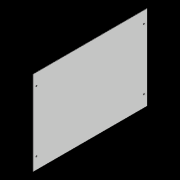
# Autodesk Inventor part: TopV4
Saved by Autodesk Inventor 2022 (Build 260153000, 153)
## iProperties
Created: 2021-10-02
Part Number: TopV4
Material: Generic
Document SubType Name: Modeling
Designer: timmy
Density: 1 g/cm^3
Appearance: Default
Author: timmy
Autodesk Inventor part; units mm, degrees
ref_plane "YZ Plane" through (0, 0, 0) normal (1, 0, 0) x (0, 1, 0)
ref_plane "XZ Plane" through (0, 0, 0) normal (0, 1, 0) x (-1, 0, 0)
ref_plane "XY Plane" through (0, 0, 0) normal (0, 0, 1) x (1, 0, 0)
sketch "Sketch1" plane through (0, 0, 0) normal (1, 0, 0) x (0, 1, 0)
  line L0 (0, 0) -> (383.54, 0)
  line L1 (383.54, 0) -> (383.54, -518.922)
  line L2 (383.54, -518.922) -> (0, -518.922)
  line L3 (0, -518.922) -> (0, 0)
  dimension "d0" = 383.54
  dimension "d1" = 518.922
  constraints: 8 end point, 2 parallel, 1 horizontal, 1 perpendicular
  measures "d0" distance of L1.end L2.end
  measures "d1" distance of L0.end L1.end
extrude "Extrusion1" add sketch "Sketch1" along normal blind 1.5875
sketch "Sketch2" plane through (1.5875, 0, 0) normal (1, 0, 0) x (0, 0, -1)
  line L0 (0, 191.77) -> (105.6706, 191.77)
  line L1 (0, 0) -> (518.922, 0) projected
  line L2 (259.461, 0) -> (259.461, 125.3156)
  line L3 (259.461, 383.54) -> (259.461, 258.2244)
  circle A0 centre (14.986, 53.4416) radius 3.175
  line L4 (518.922, 191.77) -> (413.2514, 191.77)
  circle A1 centre (503.936, 53.4416) radius 3.175
  circle A2 centre (14.986, 330.0984) radius 3.175
  circle A3 centre (503.936, 330.0984) radius 3.175
  dimension "d15" = 6.35
  constraints: 8 end point, 7 symmetric about line, 4 centre point, 1 horizontal, 1 midpoint, 1 vertical, 3 other
  measures "d15" diameter of A0
extrude "Extrusion4" cut sketch "Sketch2" against normal blind 25.4
body "Solid1"
